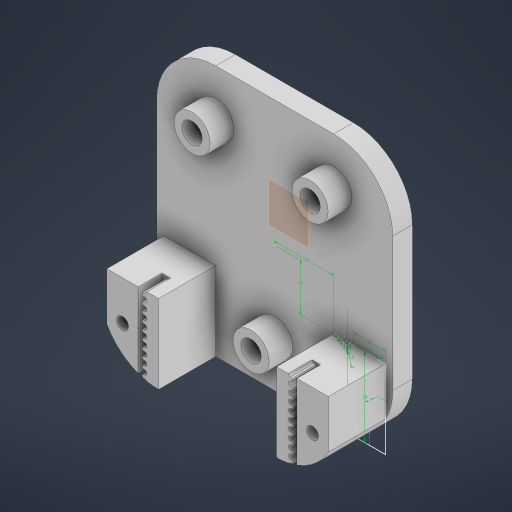
# Autodesk Inventor part: Toolhead
Saved by Autodesk Inventor 2024.2 (Build 282272000, 272)
## iProperties
Created: 2024-10-16
Part Number: Toolhead
Material: Generic
Document SubType Name: Modeling
Designer: jerem
Density: 1 g/cm^3
Appearance: Default
Author: jerem
## iProperties of the stored document Toolhead_3DPrint.ipt
Created: 2024-10-16
Part Number: Toolhead_3DPrint
Material: Generic
Document SubType Name: Modeling
Designer: jerem
Density: 1 g/cm^3
Appearance: Default
Author: jerem
Autodesk Inventor part; units mm, degrees
ref_plane "YZ Plane" through (0, 0, 0) normal (1, 0, 0) x (0, 1, 0)
ref_plane "XZ Plane" through (0, 0, 0) normal (0, 1, 0) x (-1, 0, 0)
ref_plane "XY Plane" through (0, 0, 0) normal (0, 0, 1) x (1, 0, 0)
sketch "Sketch1" plane through (0, 0, 0) normal (0, 0, 1) x (1, 0, 0)
  line L0 (0, 0) -> (0, 20.25) construction
  line L1 (0, 0) -> (0, -20.25) construction
  line L2 (0, 20.25) -> (-15, 20.25) construction
  line L3 (0, 20.25) -> (15, 20.25) construction
  circle A0 centre (-15, 20.25) radius 2.6
  circle A1 centre (15, 20.25) radius 2.6
  circle A2 centre (0, -20.25) radius 2.6
  circle A3 centre (-15, 20.25) radius 4.6
  circle A4 centre (15, 20.25) radius 4.6
  circle A5 centre (0, -20.25) radius 4.6
  circle A6 centre (-15, 20.25) radius 12 construction
  circle A7 centre (15, 20.25) radius 12 construction
  circle A8 centre (0, -20.25) radius 12 construction
  line L4 (19.8015, -9.95) -> (-19.8015, -9.95) construction
  line L5 (-19.8015, -9.95) -> (-19.8015, 9.95) construction
  line L6 (-19.8015, 9.95) -> (19.8015, 9.95) construction
  line L7 (19.8015, 9.95) -> (19.8015, -9.95) construction
  line L8 (19.8015, -9.95) -> (-19.8015, 9.95) construction
  line L9 (-19.8015, -9.95) -> (19.8015, 9.95) construction
  line L10 (-19.8015, 8.25) -> (-15, 8.25) construction
  line L11 (30, -32) -> (-30, -32)
  line L12 (-30, -32) -> (-30, 32)
  line L13 (-30, 32) -> (30, 32)
  line L14 (30, 32) -> (30, -32)
  line L15 (-30, -32) -> (30, 32) construction
  line L16 (30, -32) -> (25, -32)
  line L17 (25, -32) -> (25, -4)
  line L18 (25, -4) -> (30, -4)
  line L19 (30, -4) -> (30, -32)
  point P0 (30, -4)
  point P1 (25, -32)
  dimension "d27" = 24
  dimension "d19" = 5.2
  dimension "d20" = 5.2
  dimension "d21" = 5.2
  dimension "d22" = 2
  dimension "d23" = 2
  dimension "d24" = 2
  dimension "d25" = 40.5
  dimension "d26" = 30
  dimension "d28" = 24
  dimension "d29" = 24
  dimension "d30" = 19.9
  dimension "d43" = 60
  dimension "d44" = 64
  dimension "d60" = 28
  constraints: 40 end point, 9 coincident, 8 centre point, 6 horizontal, 6 parallel, 4 perpendicular, 3 midpoint, 2 collinear, 2 vertical, 1 point on line, 1 vertical alignment, 2 other
  measures "d19" diameter of A0
  measures "d20" diameter of A1
  measures "d21" diameter of A2
  measures "d22" radial gap between concentric circles of A3 A0
  measures "d23" radial gap between concentric circles of A4 A1
  measures "d24" radial gap between concentric circles of A5 A2
  measures "d25" distance of L1.end L0.end
  measures "d26" distance of L3.end L2.end
  measures "d28" diameter of A7
  measures "d29" diameter of A8
  measures "d30" distance of L4.end L5.end
  measures "d43" distance of L12.end L13.end
  measures "d44" distance of L11.end L12.end
  measures "d60" distance of L16.end L17.end
extrude "Extrusion1" add sketch "Sketch1" against normal blind 5 contours A3 | A4 | A5 | L11 L17 L18 L14 | L11 L12 L13 L14 L18 L17
extrude "Extrusion2" add sketch "Sketch1" along normal blind 6 contours A3 | A4 | A5
ref_plane "Work Plane1" through (15, 20.25, 11.5) normal (0, 0, 1) x (1, 0, 0)
sketch "Sketch2" plane through (0, 0, 0) normal (0, 0, 1) x (1, 0, 0)
  arc A0 (18.4573, -13.4579) -> (18, -14) centre (18.55, -14) ccw
  line L0 (18, -12) -> (15, -12)
  line L1 (18.55, -12) -> (18, -12) construction
  line L2 (15, -12) -> (15, -14)
  arc A1 (18, -12) -> (18.4573, -12.5421) centre (18.55, -12) ccw
  line L3 (18.4573, -12.5421) -> (18.9421, -12.625)
  arc A2 (19.15, -12.8714) -> (18.9421, -12.625) centre (18.9, -12.8714) ccw
  line L4 (19.15, -13) -> (18.55, -13) construction
  line L5 (19.15, -13.1286) -> (19.15, -12.8714)
  line L6 (18.9421, -13.375) -> (18.4573, -13.4579)
  line L7 (18.55, -14) -> (18.55, -12) construction
  arc A3 (18.9421, -13.375) -> (19.15, -13.1286) centre (18.9, -13.1286) ccw
  line L8 (18, -14) -> (15, -14)
  line L9 (20.15, -12) -> (20.15, -32)
  line L10 (20.15, -12) -> (28.15, -12)
  line L11 (28.15, -12) -> (28.15, -32)
  line L12 (28.15, -32) -> (20.15, -32)
  line L13 (18, -14) -> (15, -14)
  arc A4 (18, -14) -> (18.4573, -14.5421) centre (18.55, -14) ccw
  line L14 (18.4573, -14.5421) -> (18.9421, -14.625)
  line L15 (15, -14) -> (15, -16)
  line L16 (18, -16) -> (15, -16)
  line L17 (19.15, -15) -> (18.55, -15) construction
  line L18 (19.15, -15.1286) -> (19.15, -14.8714)
  line L19 (18.9421, -15.375) -> (18.4573, -15.4579)
  arc A5 (18.4573, -15.4579) -> (18, -16) centre (18.55, -16) ccw
  arc A6 (18.9421, -15.375) -> (19.15, -15.1286) centre (18.9, -15.1286) ccw
  arc A7 (19.15, -14.8714) -> (18.9421, -14.625) centre (18.9, -14.8714) ccw
  line L20 (18, -16) -> (15, -16)
  arc A8 (18, -16) -> (18.4573, -16.5421) centre (18.55, -16) ccw
  line L21 (18.4573, -16.5421) -> (18.9421, -16.625)
  line L22 (15, -16) -> (15, -18)
  line L23 (18, -18) -> (15, -18)
  line L24 (19.15, -17) -> (18.55, -17) construction
  line L25 (19.15, -17.1286) -> (19.15, -16.8714)
  line L26 (18.9421, -17.375) -> (18.4573, -17.4579)
  arc A9 (18.4573, -17.4579) -> (18, -18) centre (18.55, -18) ccw
  arc A10 (18.9421, -17.375) -> (19.15, -17.1286) centre (18.9, -17.1286) ccw
  arc A11 (19.15, -16.8714) -> (18.9421, -16.625) centre (18.9, -16.8714) ccw
  line L27 (18, -18) -> (15, -18)
  arc A12 (18, -18) -> (18.4573, -18.5421) centre (18.55, -18) ccw
  line L28 (18.4573, -18.5421) -> (18.9421, -18.625)
  line L29 (15, -18) -> (15, -20)
  line L30 (18, -20) -> (15, -20)
  line L31 (19.15, -19) -> (18.55, -19) construction
  line L32 (19.15, -19.1286) -> (19.15, -18.8714)
  line L33 (18.9421, -19.375) -> (18.4573, -19.4579)
  arc A13 (18.4573, -19.4579) -> (18, -20) centre (18.55, -20) ccw
  arc A14 (18.9421, -19.375) -> (19.15, -19.1286) centre (18.9, -19.1286) ccw
  arc A15 (19.15, -18.8714) -> (18.9421, -18.625) centre (18.9, -18.8714) ccw
  line L34 (18, -20) -> (15, -20)
  arc A16 (18, -20) -> (18.4573, -20.5421) centre (18.55, -20) ccw
  line L35 (18.4573, -20.5421) -> (18.9421, -20.625)
  line L36 (15, -20) -> (15, -22)
  line L37 (18, -22) -> (15, -22)
  line L38 (19.15, -21) -> (18.55, -21) construction
  line L39 (19.15, -21.1286) -> (19.15, -20.8714)
  line L40 (18.9421, -21.375) -> (18.4573, -21.4579)
  arc A17 (18.4573, -21.4579) -> (18, -22) centre (18.55, -22) ccw
  arc A18 (18.9421, -21.375) -> (19.15, -21.1286) centre (18.9, -21.1286) ccw
  arc A19 (19.15, -20.8714) -> (18.9421, -20.625) centre (18.9, -20.8714) ccw
  line L41 (18, -22) -> (15, -22)
  arc A20 (18, -22) -> (18.4573, -22.5421) centre (18.55, -22) ccw
  line L42 (18.4573, -22.5421) -> (18.9421, -22.625)
  line L43 (15, -22) -> (15, -24)
  line L44 (18, -24) -> (15, -24)
  line L45 (19.15, -23) -> (18.55, -23) construction
  line L46 (19.15, -23.1286) -> (19.15, -22.8714)
  line L47 (18.9421, -23.375) -> (18.4573, -23.4579)
  arc A21 (18.4573, -23.4579) -> (18, -24) centre (18.55, -24) ccw
  arc A22 (18.9421, -23.375) -> (19.15, -23.1286) centre (18.9, -23.1286) ccw
  arc A23 (19.15, -22.8714) -> (18.9421, -22.625) centre (18.9, -22.8714) ccw
  line L48 (18, -24) -> (15, -24)
  arc A24 (18, -24) -> (18.4573, -24.5421) centre (18.55, -24) ccw
  line L49 (18.4573, -24.5421) -> (18.9421, -24.625)
  line L50 (15, -24) -> (15, -26)
  line L51 (18, -26) -> (15, -26)
  line L52 (19.15, -25) -> (18.55, -25) construction
  line L53 (19.15, -25.1286) -> (19.15, -24.8714)
  line L54 (18.9421, -25.375) -> (18.4573, -25.4579)
  arc A25 (18.4573, -25.4579) -> (18, -26) centre (18.55, -26) ccw
  arc A26 (18.9421, -25.375) -> (19.15, -25.1286) centre (18.9, -25.1286) ccw
  arc A27 (19.15, -24.8714) -> (18.9421, -24.625) centre (18.9, -24.8714) ccw
  line L55 (18, -26) -> (15, -26)
  arc A28 (18, -26) -> (18.4573, -26.5421) centre (18.55, -26) ccw
  line L56 (18.4573, -26.5421) -> (18.9421, -26.625)
  line L57 (15, -26) -> (15, -28)
  line L58 (18, -28) -> (15, -28)
  line L59 (19.15, -27) -> (18.55, -27) construction
  line L60 (19.15, -27.1286) -> (19.15, -26.8714)
  line L61 (18.9421, -27.375) -> (18.4573, -27.4579)
  arc A29 (18.4573, -27.4579) -> (18, -28) centre (18.55, -28) ccw
  arc A30 (18.9421, -27.375) -> (19.15, -27.1286) centre (18.9, -27.1286) ccw
  arc A31 (19.15, -26.8714) -> (18.9421, -26.625) centre (18.9, -26.8714) ccw
  line L62 (18, -28) -> (15, -28)
  arc A32 (18, -28) -> (18.4573, -28.5421) centre (18.55, -28) ccw
  line L63 (18.4573, -28.5421) -> (18.9421, -28.625)
  line L64 (15, -28) -> (15, -30)
  line L65 (18, -30) -> (15, -30)
  line L66 (19.15, -29) -> (18.55, -29) construction
  line L67 (19.15, -29.1286) -> (19.15, -28.8714)
  line L68 (18.9421, -29.375) -> (18.4573, -29.4579)
  arc A33 (18.4573, -29.4579) -> (18, -30) centre (18.55, -30) ccw
  arc A34 (18.9421, -29.375) -> (19.15, -29.1286) centre (18.9, -29.1286) ccw
  arc A35 (19.15, -28.8714) -> (18.9421, -28.625) centre (18.9, -28.8714) ccw
  line L69 (18, -30) -> (15, -30)
  arc A36 (18, -30) -> (18.4573, -30.5421) centre (18.55, -30) ccw
  line L70 (18.4573, -30.5421) -> (18.9421, -30.625)
  line L71 (15, -30) -> (15, -32)
  line L72 (18, -32) -> (15, -32)
  line L73 (19.15, -31) -> (18.55, -31) construction
  line L74 (19.15, -31.1286) -> (19.15, -30.8714)
  line L75 (18.9421, -31.375) -> (18.4573, -31.4579)
  arc A37 (18.4573, -31.4579) -> (18, -32) centre (18.55, -32) ccw
  arc A38 (18.9421, -31.375) -> (19.15, -31.1286) centre (18.9, -31.1286) ccw
  arc A39 (19.15, -30.8714) -> (18.9421, -30.625) centre (18.9, -30.8714) ccw
  circle A40 centre (24.15, -22) radius 1.5
  line L76 (24.15, -12) -> (24.15, -32) construction
  line L77 (18, -12) -> (20.15, -12)
  line L78 (18, -32) -> (20.15, -32)
  point P0 (0, 0)
  dimension "d37" = 1.1
  dimension "d38" = 1.1
  dimension "d39" = 2
  dimension "d40" = 0.25
  dimension "d41" = -0.75
  dimension "d42" = 3
  dimension "d49" = 15
  dimension "d50" = 12
  dimension "d51" = 1.15
  dimension "d55" = 20
  dimension "d57" = 1
  dimension "d59" = 8
  dimension "d65" = 2
  dimension "d71" = 3
  constraints: 158 end point, 80 point on circle, 41 centre point, 6 perpendicular, 6 tangent, 5 midpoint, 2 horizontal, 2 line through centre, 2 vertical, 1 collinear, 1 equal radius, 1 parallel, 1 point on line, 243 other
  measures "d37" diameter of A0
  measures "d38" diameter of A1
  measures "d39" distance of L1.start L7.start
  measures "d40" radius of A3
  measures "d41" distance of L3.end L6.start
  measures "d42" distance of L1.end L0.end
  measures "d49" horizontal distance of point (0, 0) L0.end
  measures "d50" distance from line of point (0, 0) L0
  measures "d51" horizontal distance of L1.end L4.start
  measures "d55" distance of L9.start L9.end
  measures "d57" distance between parallel lines of L9 L5
  measures "d59" distance of L9.start L10.end
  measures "d65" distance of L1.start A4.centre
  measures "d71" diameter of A40
extrude "Extrusion3" add sketch "Sketch2" along normal mid plane 6 from surface at 11.5 contours A0 L8 L2 L0 A1 L3 A2 L5 A3 L6 | A4 L14 A7 L18 A6 L19 A5 L16 L15 L8 | L16 A8 L21 A11 L25 A10 L26 A9 L23 L22 | L23 A12 L28 A15 L32 A14 L33 A13 L30 L29 | L10 L11 L12 L9 | L30 A16 L35 A19 L39 A18 L40 A17 L37 L36 | L37 A20 L42 A23 L46 A22 L47 A21 L44 L43 | L72 L71 L65 A36 L70 A39 L74 A38 L75 A37 | L44 A24 L49 A27 L53 A26 L54 A25 L51 L50 | L51 A28 L56 A31 L60 A30 L61 A29 L58 L57 | L64 L58 A32 L63 A35 L67 A34 L68 A33 L65
extrude "Extrusion5" add sketch "Sketch2" along normal up to surface (8.5 mm away) contours L6 A3 L5 A2 L3 A1 L77 L9 L78 A37 L75 A38 L74 A39 L70 A36 A33 L68 A34 L67 A35 L63 A32 A29 L61 A30 L60 A31 L56 A28 A25 L54 A26 L53 A27 L49 A24 A21 L47 A22 L46 A23 L42 A20 A17 L40 A18 L39 A19 L35 A16 A13 L33 A14 L32 A15 L28 A12 A9 L26 A10 L25 A11 L21 A8 A5 L19 A6 L18 A7 L14 A4 A0 | A0 L8 L2 L0 A1 L3 A2 L5 A3 L6 | A4 L14 A7 L18 A6 L19 A5 L16 L15 L8 | L16 A8 L21 A11 L25 A10 L26 A9 L23 L22 | L23 A12 L28 A15 L32 A14 L33 A13 L30 L29 | L10 L11 L12 L9 | L30 A16 L35 A19 L39 A18 L40 A17 L37 L36 | L37 A20 L42 A23 L46 A22 L47 A21 L44 L43 | L72 L71 L65 A36 L70 A39 L74 A38 L75 A37 | L44 A24 L49 A27 L53 A26 L54 A25 L51 L50 | L51 A28 L56 A31 L60 A30 L61 A29 L58 L57 | L64 L58 A32 L63 A35 L67 A34 L68 A33 L65 | A40
mirror "Mirror1" about plane through (0, 0, 0) normal (1, 0, 0) of "Extrusion3", "Extrusion5"
fillet "Fillet1" radius 15 4 edges at (-30, 32, -2.5) (30, 32, -2.5) (-30, -32, -2.5) (30, -32, -2.5)
equation "\"d20\" = d19"
equation "\"d21\" = d19"
equation "\"d23\" = d22"
equation "\"d24\" = d22"
body "Solid1"
